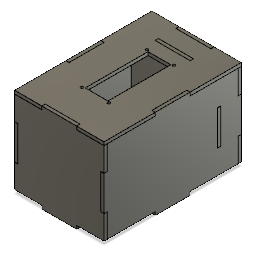
Basic Box Form_Cube for TI v2 (Autodesk Fusion 360 design; units mm, degrees)
Autodesk Fusion 360 part; units mm, degrees
sketch "Sketch1" plane through (0, 0, 0) normal (0, 1, 0) x (1, 0, 0)
  line L0 (-51.3, 78.8) -> (51.3, 78.8)
  line L1 (51.3, 78.8) -> (51.3, -78.8)
  line L2 (51.3, -78.8) -> (-51.3, -78.8)
  line L3 (-51.3, -78.8) -> (-51.3, 78.8)
  line L4 (-51.3, 78.8) -> (51.3, -78.8) construction
  line L5 (51.3, 78.8) -> (-51.3, -78.8) construction
  dimension "d1" = 157.6
  dimension "d2" = 102.6
extrude "Extrude1" add sketch "Sketch1" along normal blind 3.8 makes body 1
sketch "Sketch2" plane through (0, 3.8, 0) normal (0, 1, 0) x (-1, 0, 0)
  line L0 (51.3, 78.8) -> (-51.3, 78.8)
  line L1 (-51.3, 78.8) -> (-51.3, -78.8)
  line L2 (-51.3, -78.8) -> (51.3, -78.8)
  line L3 (51.3, -78.8) -> (51.3, 78.8)
  line L4 (51.3, -78.8) -> (-51.3, -78.8)
  line L5 (-51.3, -78.8) -> (-51.3, -75)
  line L6 (-51.3, -75) -> (51.3, -75)
  line L7 (51.3, -75) -> (51.3, -78.8)
  dimension "d5" = 3.8
  dimension "d6" = 102.6
extrude "Extrude2" add sketch "Sketch2" along normal blind 95 separate body contours L1 L2 L3 L4 L5 L6 L7 makes body 2
sketch "Sketch3" plane through (0, 98.8, 0) normal (0, 1, 0) x (-1, 0, 0)
  line L0 (51.3, -75) -> (-51.3, -75)
  line L1 (-51.3, -75) -> (-51.3, -78.8)
  line L2 (-51.3, -78.8) -> (51.3, -78.8)
  line L3 (51.3, -78.8) -> (51.3, -75)
  line L4 (20, -78.8) -> (20, -9.8696) construction
  line L5 (20, -78.8) -> (-20, -78.8)
  line L6 (-20, -78.8) -> (-20, -75)
  line L7 (-20, -75) -> (20, -75)
  line L8 (20, -75) -> (20, -78.8)
  dimension "d9" = 68.9304
  dimension "d10" = 20
  dimension "d11" = 3.8
  dimension "d12" = 40
  measures "d10" distance of origin L4
  measures "d12" distance of origin
extrude "Extrude3" add sketch "Sketch3" along normal blind 3.8 contours L0 L2 L5 L6 L7 L8 bodies 2
sketch "Sketch4" plane through (0, 98.8, 0) normal (0, 1, 0) x (-1, 0, 0)
  line L0 (20, -75) -> (20, -78.8)
  line L1 (20, -78.8) -> (51.3, -78.8)
  line L2 (51.3, -78.8) -> (51.3, -75)
  line L3 (51.3, -75) -> (20, -75)
  line L4 (20, -78.8) -> (20, -25.1124) construction
  line L5 (20, -78.8) -> (-20, -78.8)
  line L6 (-20, -78.8) -> (-20, -75)
  line L7 (-20, -75) -> (20, -75)
  line L8 (20, -75) -> (20, -78.8)
  dimension "d15" = 20
  dimension "d16" = 3.8
  dimension "d17" = 40
  measures "d15" distance of origin L4
  measures "d17" distance of origin
extrude "Extrude4" add sketch "Sketch4" against normal blind 98.8 contours L0 L5 L6 L7 L8 bodies 2
sketch "Sketch5" plane through (0, 98.8, 0) normal (0, 1, 0) x (-1, 0, 0)
  line L0 (20, -75) -> (20, -78.8)
  line L1 (20, -78.8) -> (51.3, -78.8)
  line L2 (51.3, -78.8) -> (51.3, -75)
  line L3 (51.3, -75) -> (20, -75)
  line L4 (51.3, 78.8) -> (-51.3, 78.8)
  line L5 (-51.3, 78.8) -> (-51.3, -78.8)
  line L6 (-51.3, -78.8) -> (51.3, -78.8)
  line L7 (51.3, -78.8) -> (51.3, 78.8)
extrude "Extrude5" add sketch "Sketch5" along normal blind 3.8 separate body makes body 3
ref_plane "WorkPlane1" through (0, 51.3, 75) normal (0, 0, 1) x (1, 0, 0)
sketch "Sketch6" plane through (0, 51.3, 75) normal (0, 0, 1) x (1, 0, 0)
  line L0 (20, -47.5) -> (51.3, -47.5)
  line L1 (51.3, -47.5) -> (51.3, 47.5)
  line L2 (51.3, 47.5) -> (20, 47.5)
  line L3 (20, 47.5) -> (20, 51.3)
  line L4 (20, 51.3) -> (-20, 51.3)
  line L5 (-20, 51.3) -> (-20, 47.5)
  line L6 (-20, 47.5) -> (-51.3, 47.5)
  line L7 (-51.3, 47.5) -> (-51.3, -47.5)
  line L8 (-51.3, -47.5) -> (-20, -47.5)
  line L9 (-20, -47.5) -> (-20, -51.3)
  line L10 (-20, -51.3) -> (20, -51.3)
  line L11 (20, -51.3) -> (20, -47.5)
extrude "Extrude6" add sketch "Sketch6" along normal blind 3.8 separate body makes body 4
ref_plane "WorkPlane2" through (47.5, 100.7, 0) normal (1, 0, 0) x (0, 0, -1)
sketch "Sketch7" plane through (47.5, 100.7, 0) normal (1, 0, 0) x (0, 0, -1)
  line L0 (-75, -1.9) -> (75, -1.9)
  line L1 (75, -1.9) -> (75, -96.9)
  line L2 (75, -96.9) -> (-75, -96.9)
  line L3 (-75, -96.9) -> (-75, -1.9)
  line L4 (-78.8, 1.9) -> (78.8, 1.9)
  line L5 (-20, 1.9) -> (20, 1.9)
  line L6 (20, 1.9) -> (20, -1.9)
  line L7 (20, -1.9) -> (-20, -1.9)
  line L8 (-20, -1.9) -> (-20, 1.9)
  line L9 (78.8, -100.7) -> (-78.8, -100.7)
  line L10 (-20, -100.7) -> (20, -100.7)
  line L11 (20, -100.7) -> (20, -96.9)
  line L12 (20, -96.9) -> (-20, -96.9)
  line L13 (-20, -96.9) -> (-20, -100.7)
  line L14 (-78.8, -96.9) -> (-78.8, -1.9)
  line L15 (78.8, -96.9) -> (78.8, -1.9)
  line L16 (78.8, -49.4) -> (-158.4491, -49.4) construction
  line L17 (-78.8, -29.4) -> (-75, -29.4)
  line L18 (-75, -29.4) -> (-75, -69.4)
  line L19 (-75, -69.4) -> (-78.8, -69.4)
  line L20 (-78.8, -69.4) -> (-78.8, -29.4)
  line L21 (78.8, -29.4) -> (75, -29.4)
  line L22 (75, -29.4) -> (75, -69.4)
  line L23 (75, -69.4) -> (78.8, -69.4)
  line L24 (78.8, -69.4) -> (78.8, -29.4)
  dimension "d26" = 20
  dimension "d27" = 40
  dimension "d28" = 20
  dimension "d29" = 40
  dimension "d30" = 20
  dimension "d31" = 40
  dimension "d32" = 20
  dimension "d33" = 40
  measures "d26" distance of origin
extrude "Extrude7" add sketch "Sketch7" along normal blind 3.8 separate body makes body 5
ref_plane "WorkPlane3" through (-47.5, 51.3, 0) normal (-1, 0, 0) x (0, 0, 1)
sketch "Sketch8" plane through (-47.5, 51.3, 0) normal (-1, 0, 0) x (0, 0, -1)
  line L0 (78.8, 20) -> (75, 20)
  line L1 (75, 20) -> (75, 47.5)
  line L2 (75, 47.5) -> (20, 47.5)
  line L3 (20, 47.5) -> (20, 51.3)
  line L4 (20, 51.3) -> (-20, 51.3)
  line L5 (-20, 51.3) -> (-20, 47.5)
  line L6 (-20, 47.5) -> (-75, 47.5)
  line L7 (-75, 47.5) -> (-75, 20)
  line L8 (-75, 20) -> (-78.8, 20)
  line L9 (-78.8, 20) -> (-78.8, -20)
  line L10 (-78.8, -20) -> (-75, -20)
  line L11 (-75, -20) -> (-75, -47.5)
  line L12 (-75, -47.5) -> (-20, -47.5)
  line L13 (-20, -47.5) -> (-20, -51.3)
  line L14 (-20, -51.3) -> (20, -51.3)
  line L15 (20, -51.3) -> (20, -47.5)
  line L16 (20, -47.5) -> (75, -47.5)
  line L17 (75, -47.5) -> (75, -20)
  line L18 (75, -20) -> (78.8, -20)
  line L19 (78.8, -20) -> (78.8, 20)
extrude "Extrude8" add sketch "Sketch8" along normal blind 3.8 separate body makes body 6
combine "Combine1" operation cut target body 3 tool bodies 4 6 5 2 keep tools
combine "Combine2" operation cut target body 4 tool bodies 5 6 keep tools
combine "Combine3" operation cut target body 1 tool bodies 4 6 5 2 keep tools
combine "Combine4" operation cut target body 2 tool bodies 5 6 keep tools
sketch "Sketch9" plane through (0, 102.6, 0) normal (0, 1, 0) x (-1, 0, 0)
  line L0 (20, -75) -> (20, -78.8)
  line L1 (20, -78.8) -> (51.3, -78.8)
  line L2 (51.3, -78.8) -> (51.3, -20)
  line L3 (51.3, -20) -> (47.5, -20)
  line L4 (47.5, -20) -> (47.5, 20)
  line L5 (47.5, 20) -> (51.3, 20)
  line L6 (51.3, 20) -> (51.3, 78.8)
  line L7 (51.3, 78.8) -> (20, 78.8)
  line L8 (20, 78.8) -> (20, 75)
  line L9 (20, 75) -> (-20, 75)
  line L10 (-20, 75) -> (-20, 78.8)
  line L11 (-20, 78.8) -> (-51.3, 78.8)
  line L12 (-51.3, 78.8) -> (-51.3, 20)
  line L13 (-51.3, 20) -> (-47.5, 20)
  line L14 (-47.5, 20) -> (-47.5, -20)
  line L15 (-47.5, -20) -> (-51.3, -20)
  line L16 (-51.3, -20) -> (-51.3, -78.8)
  line L17 (-51.3, -78.8) -> (-20, -78.8)
  line L18 (-20, -78.8) -> (-20, -75)
  line L19 (-20, -75) -> (20, -75)
  line L20 (-17.9, -39.85) -> (17.9, -39.85) construction
  line L21 (17.9, -39.85) -> (17.9, 39.85) construction
  line L22 (17.9, 39.85) -> (-17.9, 39.85) construction
  line L23 (-17.9, 39.85) -> (-17.9, -39.85) construction
  line L24 (-17.9, -39.85) -> (17.9, 39.85) construction
  line L25 (17.9, -39.85) -> (-17.9, 39.85) construction
  line L26 (-15.4, -44.5115) -> (-15.4, 44.2981) construction
  line L27 (15.4, -43.2428) -> (15.4, 46.0743) construction
  line L28 (-22.3225, -37.35) -> (22.0823, -37.35) construction
  line L29 (-22.3225, 37.35) -> (26.6497, 37.35) construction
  circle A0 centre (-15.4, 37.35) radius 1.5
  circle A1 centre (15.4, 37.35) radius 1.5
  circle A2 centre (-15.4, -37.35) radius 1.5
  circle A3 centre (15.4, -37.35) radius 1.5
  line L30 (13, -36) -> (-13, -36)
  line L31 (-13, -36) -> (-13, 36)
  line L32 (-13, 36) -> (13, 36)
  line L33 (13, 36) -> (13, -36)
  line L34 (13, -36) -> (-13, 36) construction
  line L35 (-13, -36) -> (13, 36) construction
  dimension "d39" = 79.7
  dimension "d40" = 35.8
  dimension "d41" = 2.5
  dimension "d42" = 2.5
  dimension "d43" = 2.5
  dimension "d44" = 2.5
  dimension "d45" = 3
  dimension "d46" = 3
  dimension "d47" = 3
  dimension "d48" = 3
  dimension "d49" = 26
  dimension "d50" = 72
  measures "d41" distance of L23 L26
  measures "d42" distance of L21 L27
  measures "d43" distance of L20 L28
  measures "d44" distance of L22 L29
  measures "d45" diameter of A0
  measures "d46" diameter of A1
  measures "d47" diameter of A2
  measures "d48" diameter of A3
extrude "Extrude9" cut sketch "Sketch9" against normal blind 4 contours A0 | A1 | A2 | A3 | L30 L31 L32 L33 bodies 3
ref_plane "WorkPlane4" through (0, 51.3, -55) normal (0, 0, 1) x (1, 0, 0)
sketch "Sketch10" plane through (0, 51.3, -55) normal (0, 0, 1) x (1, 0, 0)
  line L0 (-47.5, 20) -> (-47.5, -20)
  line L1 (-47.5, -20) -> (-51.3, -20)
  line L2 (-51.3, -20) -> (-51.3, -47.5)
  line L3 (-51.3, -47.5) -> (-20, -47.5)
  line L4 (-20, -47.5) -> (-20, -51.3)
  line L5 (-20, -51.3) -> (20, -51.3)
  line L6 (20, -51.3) -> (20, -47.5)
  line L7 (20, -47.5) -> (51.3, -47.5)
  line L8 (51.3, -47.5) -> (51.3, -20)
  line L9 (51.3, -20) -> (47.5, -20)
  line L10 (47.5, -20) -> (47.5, 20)
  line L11 (47.5, 20) -> (51.3, 20)
  line L12 (51.3, 20) -> (51.3, 47.5)
  line L13 (51.3, 47.5) -> (20, 47.5)
  line L14 (20, 47.5) -> (20, 51.3)
  line L15 (20, 51.3) -> (-20, 51.3)
  line L16 (-20, 51.3) -> (-20, 47.5)
  line L17 (-20, 47.5) -> (-51.3, 47.5)
  line L18 (-51.3, 47.5) -> (-51.3, 20)
  line L19 (-51.3, 20) -> (-47.5, 20)
extrude "Extrude10" add sketch "Sketch10" along normal blind 3.8 separate body makes body 7
extrude "Extrude11" add 1 faces at (47.5, 44.6333, -53.7333) along direction (1, 0, 0) blind 7.6 on bodies 7 bodies 7
extrude "Extrude12" add 1 faces at (-47.5, 57.9667, -53.7333) along direction (-1, 0, 0) blind 7.6 on bodies 7 bodies 7
extrude "Extrude13" cut 2 faces at (51.3, 80.4667, -52.4667) (51.3, 12.9667, -52.4667) along direction (-1, 0, 0) blind 3.8 on bodies 7 bodies 7
extrude "Extrude14" cut 2 faces at (-51.3, 89.6333, -52.4667) (-51.3, 22.1333, -52.4667) along direction (1, 0, 0) blind 3.8 on bodies 7 bodies 7
extrude "Extrude15" cut 1 faces at (55.1, 44.6333, -53.7333) along direction (-1, 0, 0) blind 3.8 on bodies 7 bodies 7
extrude "Extrude16" cut 1 faces at (-55.1, 57.9667, -53.7333) along direction (1, 0, 0) blind 3.8 on bodies 7 bodies 7
combine "Combine5" operation cut target body 6 tool bodies 7 5 keep tools
hidden bodies 1
equation "d1 = ( 3.8 * 2 ) * 1 mm + 150 mm"
equation "d2 = 95 mm + 7.60 mm"
equation "d6 = 95 mm + 7.60 mm"
equation "d18 = -95 mm - 3.8 mm"
equation "d56 = ( 2 * 3.8 ) * 1 mm"
equation "d58 = 2 * 3.8000 mm"
